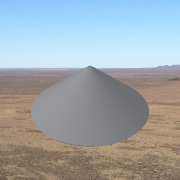
# Autodesk Inventor part: chimneyCap
Saved by Autodesk Inventor 2014 SP1 (Build 180222100, 222)
## iProperties
Created: 2014-05-22
Part Number: chimneyCap
Material: Generic
Document SubType Name: Modeling
Designer: Dave
Density: 1 g/cm^3
Appearance: Default
Author: Dave
Autodesk Inventor part; units mm, degrees
ref_plane "YZ Plane" through (0, 0, 0) normal (1, 0, 0) x (0, 1, 0)
ref_plane "XZ Plane" through (0, 0, 0) normal (0, 1, 0) x (-1, 0, 0)
ref_plane "XY Plane" through (0, 0, 0) normal (0, 0, 1) x (1, 0, 0)
sketch "Sketch1" plane through (0, 0, 0) normal (1, 0, 0) x (0, 1, 0)
  line L0 (-141.3585, 145.9726) -> (-136.7969, 150.3901)
  line L1 (-136.7969, 150.3901) -> (4.5616, 4.4175)
  line L2 (4.5616, 4.4175) -> (0, 0)
  line L3 (0, 0) -> (-141.3585, 145.9726)
  line L4 (-170.5426, 0) -> (33.7457, 0) projected
  point P0 (0, 0)
  dimension "d0" = 6.35
  dimension "d1" = 203.2
  constraints: 8 end point, 2 parallel, 1 perpendicular
  measures "d0" distance of L1.end L2.end
  measures "d1" distance of L0.end L1.end
revolve "Revolution1" add sketch "Sketch1" angle 360 about axis through (0, -10, 0) along (0, 1, 0)
body "Solid1"
